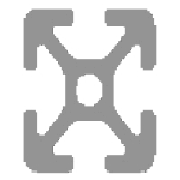
# Autodesk Inventor part: Generic-1
Saved by Autodesk Inventor 2020 (Build 240168000, 168)
## iProperties
Created: 2020-04-09
Part Number: Generic-1
Material: Generic
Document SubType Name: Modeling
Standard: Unnamed
Designer: Simon
Language: en-US
Size Designation: Generic-1
Categories: <MemberInstance><Categories><Category DisplayName="Structural Shapes" InternalName="089c4875-fa83-4c05-b084-43b9cc11f5ed" Mnemonic="GRDR"><CategoryParameter DisplayName="Mass per Length Unit" InternalName="0bb95a10-148f-4027-a459-38d7b056702a" Mnemonic="shpmass"/><CategoryParameter DisplayName="Section Area" InternalName="1ff91680-64b0-4202-b9a3-7fd3f94bba3b" Mnemonic="secarea"/><CategoryParameter DisplayName="Radius of Gyration (x)" InternalName="25778675-03e9-40c1-b6a8-4a9ed693320d" Mnemonic="gyrradx"/><CategoryParameter DisplayName="Torsional Rigidity Modulus" InternalName="26c1ec35-5026-4c63-ad0a-751cf684a536" Mnemonic="torrigmod"/><CategoryParameter DisplayName="Distance of the Center of Gravity X-X" InternalName="26c9bdb8-9c79-4b4f-a92e-8e197583c9c4" Mnemonic="grcendistX"/><CategoryParameter DisplayName="Legacy Member ID" InternalName="340afe4f-75d7-48d3-ab7d-943f3c3da468" Mnemonic="LegacyMemberID"/><CategoryParameter DisplayName="Base Length" InternalName="42e34263-8f20-4d0e-ad48-bf1385b87c24" Mnemonic="shplen"/><CategoryParameter DisplayName="Moment of Inertia (y)" InternalName="4b9f58ea-bced-460e-81ea-3d29ca5a49e3" Mnemonic="inermomy"/><CategoryParameter DisplayName="Moment of Inertia (x)" InternalName="4cd780bc-73d7-43ac-917a-579e5cbd684d" Mnemonic="inermomx"/><CategoryParameter DisplayName="Custom Base Point" InternalName="4f1d1b73-316d-484b-a3df-9cbabb16eb77" Mnemonic="shpBasePoint"/><CategoryParameter DisplayName="Shape Height" InternalName="50274e7d-5ac0-4796-92cb-c59e54983c67" Mnemonic="shpheig"/><CategoryParameter DisplayName="Section Module (y)" InternalName="59eaa5e9-d227-48dc-b6c1-6920f96e0f95" Mnemonic="secmody"/><CategoryParameter DisplayName="Section Designation" InternalName="5a64d034-428d-49c8-ba32-7619764de20f" Mnemonic="shpdes"/><CategoryParameter DisplayName="Section Module (x)" InternalName="72cfad18-cf51-4ed4-aaa7-c6b224f8419f" Mnemonic="secmodx"/><CategoryParameter DisplayName="Torsional Section Modulus" InternalName="7c55a8dc-8844-49f9-a867-cc677b30ec9a" Mnemonic="torsecmod"/><CategoryParameter DisplayName="Shape Width" InternalName="7c717d54-a18f-4666-b4d4-573cce22c62c" Mnemonic="shpwdth"/><CategoryParameter DisplayName="Second Shape Thickness" InternalName="9251a8e1-85fd-4e47-af99-afdb762317d9" Mnemonic="shpthick2"/><CategoryParameter DisplayName="FG Authored" InternalName="9c666724-f362-4ea7-ac62-f6a007de5c69" Mnemonic="shpFGAuto"/><CategoryParameter DisplayName="Distance of the Center of Gravity Y-Y" InternalName="bcc4fb17-7af4-436a-8f8c-d0aa3b0248c5" Mnemonic="grcendistY"/><CategoryParameter DisplayName="Radius of Gyration (y)" InternalName="bfa18ebe-1636-4dbe-8d42-b263e0b73184" Mnemonic="gyrrady"/><CategoryParameter DisplayName="Shape Thickness" InternalName="d109cf76-8eb4-42fc-9800-4409734adc67" Mnemonic="shpthick"/><CategoryParameter DisplayName="Coefficient of Shear Displacement" InternalName="de4c90c6-aaa8-468f-a335-6737b311b5d3" Mnemonic="shdispc"/><Category DisplayName="Other" InternalName="f02205ff-2390-476f-921c-0b3185f88e84" Mnemonic="OTHSHP"><CategoryParameter DisplayName="Moment of Inertia (y)" InternalName="044c654e-f649-48ac-84cc-650a29ae31ca" Mnemonic="inermomy"/><CategoryParameter DisplayName="Shape Thickness" InternalName="12b1a788-9233-48fd-a933-2df8ff42b15f" Mnemonic="shpthick"/><CategoryParameter DisplayName="Mass per Length Unit" InternalName="2fd289d6-9394-4d2d-97e6-6659d7d4551d" Mnemonic="shpmass"/><CategoryParameter DisplayName="Radius of Gyration (y)" InternalName="743e1dfe-1bba-408b-b985-cf752b207386" Mnemonic="gyrrady"/><CategoryParameter DisplayName="Section Module (y)" InternalName="88b8bff9-a616-4028-93d5-ed4f79680d13" Mnemonic="secmody"/><CategoryParameter DisplayName="Section Area" InternalName="c46ecdf8-b6eb-4db9-8b25-30258930c1e3" Mnemonic="secarea"/><CategoryParameter DisplayName="Section Module (x)" InternalName="cac70804-9d39-43bb-be17-56ea1f39a6c2" Mnemonic="secmodx"/><CategoryParameter DisplayName="Moment of Inertia (x)" InternalName="ec6737bc-264f-43ed-b0bd-f6d410c2718d" Mnemonic="inermomx"/><CategoryParameter DisplayName="Radius of Gyration (x)" InternalName="ee72c61e-565e-4fd6-b448-66e1e1abcb7e" Mnemonic="gyrradx"/></Category></Category><Category DisplayName="DataType" InternalName="23b78d0f-2648-40c6-8793-ca6db495c9e8" Mnemonic="DATATYPE"><CategoryParameter DisplayName="DisplayName" InternalName="05415f3d-3907-474b-a020-eb9d644f4cf3" Mnemonic="DISPLAYNAME"/><CategoryParameter DisplayName="Standard" InternalName="0c0a119c-1e12-4c84-803f-101930972f5e" Mnemonic="STANDARD"/><CategoryParameter DisplayName="Description" InternalName="13903e3d-64b1-4950-80da-f627842ea37f" Mnemonic="DESCRIPTION"/><CategoryParameter DisplayName="Designation" InternalName="2675968c-4ce5-49e0-a4f5-552d29089031" Mnemonic="DESIGNATION"/><CategoryParameter DisplayName="Default Row" InternalName="2af9ec52-faaa-4026-b378-f9fa4afca842" Mnemonic="DEFAULTROW"/><CategoryParameter DisplayName="Folder Name" InternalName="3f06958e-8713-4116-9be7-ed6184ecc97b" Mnemonic="FOLDERNAME"/><CategoryParameter DisplayName="Revision Guid" InternalName="45a75005-10b1-4dfc-8d6d-dfe629f0b93c" Mnemonic="REVISIONGUID"/><CategoryParameter DisplayName="FileName" InternalName="8b46a4cc-9585-4fed-90c3-899f57e09a73" Mnemonic="FILENAME"/><CategoryParameter DisplayName="StdsOrg" InternalName="8f5914e1-4693-403f-8ab5-d37768198c9d" Mnemonic="STDSORG"/><CategoryParameter DisplayName="Family Version" InternalName="914462f6-6e19-4b14-ba84-155b9680b1d0" Mnemonic="FAMILYREVISION"/><CategoryParameter DisplayName="Standard Revision" InternalName="91d5a463-65c2-4fde-b823-3b7fea5e8e17" Mnemonic="STANDARDREVISION"/><CategoryParameter DisplayName="Member Revision" InternalName="a65d44b9-392f-4f4f-857b-e4b3d54996fe" Mnemonic="MEMBERREVISION"/><CategoryParameter DisplayName="ClipFormat" InternalName="bc51e27b-3422-4e78-93ef-cec197ddf230" Mnemonic="CLIPFORMAT"/><CategoryParameter DisplayName="Manufacturer" InternalName="cd6c7a72-a28a-4e50-99a9-2c7f4e13e5ad" Mnemonic="MANUFACTURER"/><CategoryParameter DisplayName="InternalName" InternalName="cf1d0246-76d9-4b4a-8305-fa0409afb5c1" Mnemonic="INTERNALNAME"/><CategoryParameter DisplayName="IsMetric" InternalName="e2385c5b-1ea4-4823-96a8-8de651266ec3" Mnemonic="ISMETRIC"/><Category DisplayName="Part" InternalName="c0e0b642-3bcb-4cc8-9e80-f96d35c4afa4" Mnemonic="PART"><CategoryParameter DisplayName="Part Number" InternalName="016b6077-bfbe-49bd-92c9-d8d59c39c941" Mnemonic="PARTNUMBER"/><CategoryParameter DisplayName="Stock Number" InternalName="4dba7c1c-e26c-444e-836c-b08b433409a8" Mnemonic="STOCKNUMBER"/><CategoryParameter DisplayName="Material Key" InternalName="5c9a8adb-dd2b-4535-b97f-0a94a95fe41f" Mnemonic="MATERIALKEY"/><CategoryParameter DisplayName="Material" InternalName="818a152a-d3c3-49ca-80ee-df7d91421b8e" Mnemonic="MATERIAL"/></Category></Category></Categories><FamilyTemplate Id="Extruson profile"><FamilyTemplateParameters><FamilyTemplateParameter ObjectType="kModelParameterObject" ValueType="xs:double" Id="12" ObjectReferenceKey="length"/><FamilyTemplateParameter ObjectType="kPartComponentDefinitionObject" ValueType="xs:string" Id="23" SubObjectId="Material"/><FamilyTemplateParameter ObjectType="kPropertyObject" ValueType="xs:string" Id="26" ObjectReferenceKey="{32853F0F-3444-11d1-9E93-0060B03C1CA6}" SubObjectId="5"/><FamilyTemplateParameter ObjectType="kPropertyObject" ValueType="xs:string" Id="27" ObjectReferenceKey="{32853F0F-3444-11d1-9E93-0060B03C1CA6}" SubObjectId="52"/></FamilyTemplateParameters></FamilyTemplate><CategoryParameterMap><ParamToTemplateMap><ParamToTemplate CategoryParameter="//CategoryParameter[@InternalName='cf1d0246-76d9-4b4a-8305-fa0409afb5c1']" ConstantValue="46895b43-b019-4b51-a2ac-e50d46f6f880"/><ParamToTemplate CategoryParameter="//CategoryParameter[@InternalName='45a75005-10b1-4dfc-8d6d-dfe629f0b93c']" ConstantValue="6d3aefb0-d34e-4c6a-b983-9b6ad091efc6"/><ParamToTemplate CategoryParameter="//CategoryParameter[@InternalName='3f06958e-8713-4116-9be7-ed6184ecc97b']" ConstantValue="Extrusion Profile"/><ParamToTemplate CategoryParameter="//CategoryParameter[@InternalName='8f5914e1-4693-403f-8ab5-d37768198c9d']" TemplateParameter="17"/><ParamToTemplate CategoryParameter="//CategoryParameter[@InternalName='0c0a119c-1e12-4c84-803f-101930972f5e']" TemplateParameter="18"/><ParamToTemplate CategoryParameter="//CategoryParameter[@InternalName='91d5a463-65c2-4fde-b823-3b7fea5e8e17']" TemplateParameter="19"/><ParamToTemplate CategoryParameter="//CategoryParameter[@InternalName='cd6c7a72-a28a-4e50-99a9-2c7f4e13e5ad']" TemplateParameter="20"/><ParamToTemplate CategoryParameter="//CategoryParameter[@InternalName='13903e3d-64b1-4950-80da-f627842ea37f']" TemplateParameter="22"/><ParamToTemplate CategoryParameter="//CategoryParameter[@InternalName='05415f3d-3907-474b-a020-eb9d644f4cf3']" ConstantValue="Extrusion Profile"/><ParamToTemplate CategoryParameter="//CategoryParameter[@InternalName='914462f6-6e19-4b14-ba84-155b9680b1d0']" ConstantValue="11"/><ParamToTemplate CategoryParameter="//CategoryParameter[@InternalName='bc51e27b-3422-4e78-93ef-cec197ddf230']" ConstantValue="CF_INVENTOR.STDPARTS"/><ParamToTemplate CategoryParameter="//CategoryParameter[@InternalName='e2385c5b-1ea4-4823-96a8-8de651266ec3']" ConstantValue="false"/><ParamToTemplate CategoryParameter="//CategoryParameter[@InternalName='2af9ec52-faaa-4026-b378-f9fa4afca842']" ConstantValue="1"/><ParamToTemplate CategoryParameter="//CategoryParameter[@InternalName='9c666724-f362-4ea7-ac62-f6a007de5c69']" ConstantValue="1"/><ParamToTemplate CategoryParameter="//CategoryParameter[@InternalName='8b46a4cc-9585-4fed-90c3-899f57e09a73']" ConstantValue="Generic-1-Generic-1"/><ParamToTemplate CategoryParameter="//CategoryParameter[@InternalName='a65d44b9-392f-4f4f-857b-e4b3d54996fe']" ConstantValue="5b8087e4-338b-4968-8476-bc2d84e69437"/><ParamToTemplate CategoryParameter="//CategoryParameter[@InternalName='a65d44b9-392f-4f4f-857b-e4b3d54996fe']" ConstantValue="5b8087e4-338b-4968-8476-bc2d84e69437"/><ParamToTemplate CategoryParameter="//CategoryParameter[@InternalName='2675968c-4ce5-49e0-a4f5-552d29089031']" TemplateParameter="27"/><ParamToTemplate CategoryParameter="//CategoryParameter[@InternalName='818a152a-d3c3-49ca-80ee-df7d91421b8e']" TemplateParameter="23"/><ParamToTemplate CategoryParameter="//CategoryParameter[@InternalName='016b6077-bfbe-49bd-92c9-d8d59c39c941']" TemplateParameter="26"/><ParamToTemplate CategoryParameter="//CategoryParameter[@InternalName='42e34263-8f20-4d0e-ad48-bf1385b87c24']" TemplateParameter="12"/></ParamToTemplateMap></CategoryParameterMap></MemberInstance>
Density: 1 g/cm^3
Appearance: Default
_CCFamilyDisplayName: Extrusion Profile -
_FrameMemberDoc: Frame Member File
_Version: 15.0.0
_GetPNFromCC: 1
G_L: 5.138 in
G_W: 0.787 in
G_H: 0.787 in
IsCustomPart: 1
Author: Simon
Autodesk Inventor part; units mm, degrees
ref_plane "XZ Plane" through (0, 0, 0) normal (0, 1, 0) x (-1, 0, 0)
ref_plane "Start Plane" through (20, 0, 0) normal (1, 0, 0) x (0, 1, 0)
ref_plane "End Plane" through (150.5, 0, 0) normal (1, 0, 0) x (0, 1, 0)
sketch "Sketch" plane through (0, 0, 0) normal (1, 0, 0) x (0, 1, 0)
  circle A0 centre (-3.0533, 11.4582) radius 2.1463
  line L0 (2.4543, 4.6976) -> (0.1995, 6.9525)
  arc A1 (1.8616, 3.2667) -> (2.4543, 4.6976) centre (1.8616, 4.1049) ccw
  line L1 (-0.2466, 3.2667) -> (1.8616, 3.2667)
  arc A2 (-0.2466, 3.2667) -> (-0.5514, 2.9619) centre (-0.2466, 2.9619) ccw
  line L2 (-0.5514, 2.2507) -> (-0.5514, 2.9619)
  arc A3 (-0.5514, 2.2507) -> (0.236, 1.4633) centre (0.236, 2.2507) ccw
  line L3 (4.935, 1.4633) -> (0.236, 1.4633)
  arc A4 (4.935, 1.4633) -> (6.9416, 3.4699) centre (4.935, 3.4699) ccw
  line L4 (6.9416, 8.1689) -> (6.9416, 3.4699)
  arc A5 (6.9416, 8.1689) -> (6.1542, 8.9563) centre (6.1542, 8.1689) ccw
  line L5 (5.443, 8.9563) -> (6.1542, 8.9563)
  arc A6 (5.443, 8.9563) -> (5.1382, 8.6515) centre (5.443, 8.6515) ccw
  line L6 (5.1382, 6.5433) -> (5.1382, 8.6515)
  arc A7 (3.7073, 5.9506) -> (5.1382, 6.5433) centre (4.3, 6.5433) ccw
  line L7 (1.4525, 8.2055) -> (3.7073, 5.9506)
  arc A8 (0.5746, 10.3248) -> (1.4525, 8.2055) centre (3.5718, 10.3248) ccw
  line L8 (0.5746, 12.5917) -> (0.5746, 10.3248)
  arc A9 (1.4525, 14.711) -> (0.5746, 12.5917) centre (3.5718, 12.5917) ccw
  line L9 (3.7073, 16.9658) -> (1.4525, 14.711)
  arc A10 (5.1382, 16.3731) -> (3.7073, 16.9658) centre (4.3, 16.3731) ccw
  line L10 (5.1382, 14.2649) -> (5.1382, 16.3731)
  arc A11 (5.1382, 14.2649) -> (5.443, 13.9601) centre (5.443, 14.2649) ccw
  line L11 (6.1542, 13.9601) -> (5.443, 13.9601)
  arc A12 (6.1542, 13.9601) -> (6.9416, 14.7475) centre (6.1542, 14.7475) ccw
  line L12 (6.9416, 19.4465) -> (6.9416, 14.7475)
  arc A13 (6.9416, 19.4465) -> (4.935, 21.4531) centre (4.935, 19.4465) ccw
  line L13 (0.236, 21.4531) -> (4.935, 21.4531)
  arc A14 (0.236, 21.4531) -> (-0.5514, 20.6657) centre (0.236, 20.6657) ccw
  line L14 (-0.5514, 19.9545) -> (-0.5514, 20.6657)
  arc A15 (-0.5514, 19.9545) -> (-0.2466, 19.6497) centre (-0.2466, 19.9545) ccw
  line L15 (1.8616, 19.6497) -> (-0.2466, 19.6497)
  arc A16 (2.4543, 18.2188) -> (1.8616, 19.6497) centre (1.8616, 18.8115) ccw
  line L16 (0.1995, 15.964) -> (2.4543, 18.2188)
  arc A17 (-1.9199, 15.0861) -> (0.1995, 15.964) centre (-1.9199, 18.0833) ccw
  line L17 (-4.1867, 15.0861) -> (-1.9199, 15.0861)
  arc A18 (-6.306, 15.964) -> (-4.1867, 15.0861) centre (-4.1867, 18.0833) ccw
  line L18 (-8.5609, 18.2188) -> (-6.306, 15.964)
  arc A19 (-7.9682, 19.6497) -> (-8.5609, 18.2188) centre (-7.9682, 18.8115) ccw
  line L19 (-5.86, 19.6497) -> (-7.9682, 19.6497)
  arc A20 (-5.86, 19.6497) -> (-5.5552, 19.9545) centre (-5.86, 19.9545) ccw
  line L20 (-5.5552, 20.6657) -> (-5.5552, 19.9545)
  arc A21 (-5.5552, 20.6657) -> (-6.3426, 21.4531) centre (-6.3426, 20.6657) ccw
  line L21 (-11.0416, 21.4531) -> (-6.3426, 21.4531)
  arc A22 (-11.0416, 21.4531) -> (-13.0482, 19.4465) centre (-11.0416, 19.4465) ccw
  line L22 (-13.0482, 14.7475) -> (-13.0482, 19.4465)
  arc A23 (-13.0482, 14.7475) -> (-12.2608, 13.9601) centre (-12.2608, 14.7475) ccw
  line L23 (-11.5496, 13.9601) -> (-12.2608, 13.9601)
  arc A24 (-11.5496, 13.9601) -> (-11.2448, 14.2649) centre (-11.5496, 14.2649) ccw
  line L24 (-11.2448, 16.3731) -> (-11.2448, 14.2649)
  arc A25 (-9.8139, 16.9658) -> (-11.2448, 16.3731) centre (-10.4066, 16.3731) ccw
  line L25 (-7.559, 14.711) -> (-9.8139, 16.9658)
  arc A26 (-6.6812, 12.5917) -> (-7.559, 14.711) centre (-9.6784, 12.5917) ccw
  line L26 (-6.6812, 10.3248) -> (-6.6812, 12.5917)
  arc A27 (-7.559, 8.2055) -> (-6.6812, 10.3248) centre (-9.6784, 10.3248) ccw
  line L27 (-9.8139, 5.9506) -> (-7.559, 8.2055)
  arc A28 (-11.2448, 6.5433) -> (-9.8139, 5.9506) centre (-10.4066, 6.5433) ccw
  line L28 (-11.2448, 8.6515) -> (-11.2448, 6.5433)
  arc A29 (-11.2448, 8.6515) -> (-11.5496, 8.9563) centre (-11.5496, 8.6515) ccw
  line L29 (-12.2608, 8.9563) -> (-11.5496, 8.9563)
  arc A30 (-12.2608, 8.9563) -> (-13.0482, 8.1689) centre (-12.2608, 8.1689) ccw
  line L30 (-13.0482, 3.4699) -> (-13.0482, 8.1689)
  arc A31 (-13.0482, 3.4699) -> (-11.0416, 1.4633) centre (-11.0416, 3.4699) ccw
  line L31 (-6.3426, 1.4633) -> (-11.0416, 1.4633)
  arc A32 (-6.3426, 1.4633) -> (-5.5552, 2.2507) centre (-6.3426, 2.2507) ccw
  line L32 (-5.5552, 2.9619) -> (-5.5552, 2.2507)
  arc A33 (-5.5552, 2.9619) -> (-5.86, 3.2667) centre (-5.86, 2.9619) ccw
  line L33 (-7.9682, 3.2667) -> (-5.86, 3.2667)
  arc A34 (-8.5609, 4.6976) -> (-7.9682, 3.2667) centre (-7.9682, 4.1049) ccw
  line L34 (-6.306, 6.9525) -> (-8.5609, 4.6976)
  arc A35 (-4.1867, 7.8303) -> (-6.306, 6.9525) centre (-4.1867, 4.8331) ccw
  line L35 (-1.9199, 7.8303) -> (-4.1867, 7.8303)
  arc A36 (0.1995, 6.9525) -> (-1.9199, 7.8303) centre (-1.9199, 4.8331) ccw
  point P0 (0, 0)
  constraints: 72 end point, 72 point on circle, 37 centre point
extrude "Body" add sketch "Sketch" along normal up to surface (130.5 mm away) from surface at 20
sketch "Sketch2" plane through (0, 0, 0) normal (1, 0, 0) x (0, 1, 0)
  line L0 (0, 0) -> (10, 0)
ref_plane "Work Plane3" through (0, 0, 0) normal (0, 0, -1) x (0, 1, 0)
sketch "Sketch3" plane through (0, 0, 0) normal (0, 0, -1) x (0, 1, 0)
  line L0 (-2, 20) -> (12, 20)
  line L1 (-2, 150.5) -> (12, 150.5)
  dimension "d7" = 130.5
  measures "d7" distance between parallel lines of L0 L1
equation "\"G_OFFSET_START\" = -20"
equation "\"G_OFFSET_END\" = -20"
equation "\"d2\" = -G_OFFSET_START"
equation "\"d3\" = length + G_OFFSET_END"
equation "\"G_L\" = d7"
equation "\"length\" = 170.5"
body "Solid1"
